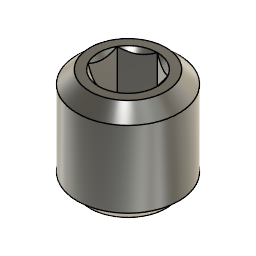
M3 Parametric Set Screw (Autodesk Fusion 360 design; units mm, degrees)
part number: M3x4mm Setscrew
Autodesk Fusion 360 part; units mm, degrees
note: some values were not read from the file. Set by a fixed rule: which sketch regions a step uses.
sketch "Sketch2" plane through (0, 0, 0) normal (1, 0, 0) x (0, 1, 0)
  line L0 (-1.5, -2.625) -> (-1.125, -3)
  line L1 (-1.125, -3) -> (0, -3)
  line L2 (0, -3) -> (0, 0)
  line L3 (-1.5, -0.375) -> (-1.5, -2.625)
  line L4 (0, 0) -> (-1.125, 0)
  line L5 (-0.866, 0) -> (0, -0.866)
  line L6 (-1.125, 0) -> (-1.5, -0.375)
  point P0 (-1.75, 2)
  point P1 (-1.5, 0)
  dimension "d24" = 1.5
  dimension "d25" = 45
  dimension "d26" = 0.375
  dimension "d36" = 3
  dimension "d37" = 45
  dimension "d38" = 0.866
  dimension "d42" = 0.375
  constraint perpendicular L1 L3
  constraint coincident L2.end L4.start
  constraint vertical L2
  constraint perpendicular L3 L4
  constraint coincident L4 L5.start
  constraint coincident L2 L5.end
  constraint coincident P1 L4
  constraint coincident P1 L3
  constraint vertical L0.end L4.end
  measures "d24" distance of L2 L3
  measures "d25" angle of L0 L3
  measures "d26" distance of L0.end L3
  measures "d36" distance of L2.end L1.end
  measures "d37" angle of L2 L5
  measures "d38" distance of L2.end L5.start
  measures "d42" vertical distance of L4.end L3.start
revolve "Revolve1" add sketch "Sketch2" angle 360 about axis through (0, 0, -3) along (0, 0, 1) contours L0 L1 L2 L3 L4 L5 L6
sketch "Sketch3" plane through (0, 0, 0) normal (0, 0, 1) x (1, 0, 0)
  line L0 (0.75, 0.433) -> (0, 0.866)
  line L1 (0, 0.866) -> (-0.75, 0.433)
  line L2 (-0.75, 0.433) -> (-0.75, -0.433)
  line L3 (-0.75, -0.433) -> (0, -0.866)
  line L4 (0, -0.866) -> (0.75, -0.433)
  line L5 (0.75, -0.433) -> (0.75, 0.433)
  dimension "d31" = 0.75
  constraint vertical L5
  measures "d31" distance of origin L5
extrude "Extrude4" cut sketch "Sketch3" against normal blind 1.5
equation "Length = 3 mm"
equation "d36 = Length"
equation "d38 = 1.732 mm / 2"
equation "d42 = d26"
